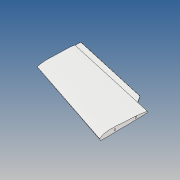
# Autodesk Inventor part: wing_r
Saved by Autodesk Inventor 2019.4 (Build 234330000, 330)
## iProperties
Part Number: wing_r
Material: GEDA Polyamid
Document SubType Name: Modeling
Designer: Admin
Density: 1.14 g/cm^3
Appearance: GEDA Polyamid A
Mass: 6967.25 g
Surface Area: 6132.4 cm^2
Volume: 6111.62 cm^3
Gewicht: 6,967 kg
G_L: 0
G_H: 0
G_B: 0
InventorVersion: 2019.4
VAULT_Status: in Bearbeitung
Revision: -
Max. Breite: 0
Max. Höhe: 0
Max. Länge: 0
Max. Abmessungen: 0 x 0 x 0
Author: Admin
Autodesk Inventor part; units mm, degrees
note: some values were not read from the file. Left out: dimensions or parameters whose unit could not be read.
ref_plane "XZ Plane" through (0, 0, 0) normal (0, 1, 0) x (-1, 0, 0)
ref_plane "XY Plane" through (0, 0, 0) normal (0, 0, 1) x (1, 0, 0)
sketch "Skizze1" plane through (0, 0, 0) normal (1, 0, 0) x (0, 1, 0)
  line L0 (190, 0) -> (-190, 0) construction
  line L1 (190, 4) -> (190, -4)
  arc A0 (-187.5, 0) -> (-191.5, -2) centre (-190, 0) ccw
  line L2 (175, 4) -> (175, -4) construction
  line L3 (160, 4) -> (160, -4) construction
  line L4 (145, 4) -> (145, -4) construction
  line L5 (130, 4) -> (130, -4) construction
  line L6 (115, 4) -> (115, -4) construction
  line L7 (100, 4) -> (100, -4) construction
  line L8 (85, 4) -> (85, -4) construction
  line L9 (70, 4) -> (70, -4) construction
  line L10 (55, 4) -> (55, -4) construction
  line L11 (40, 4) -> (40, -4) construction
  line L12 (25, 4) -> (25, -4) construction
  line L13 (10, 4) -> (10, -4) construction
  line L14 (-5, 4) -> (-5, -4) construction
  line L15 (-20, 4) -> (-20, -4) construction
  line L16 (-35, 4) -> (-35, -4) construction
  line L17 (-50, 4) -> (-50, -4) construction
  line L18 (-65, 4) -> (-65, -4) construction
  line L19 (-80, 4) -> (-80, -4) construction
  line L20 (-95, 4) -> (-95, -4) construction
  line L21 (-110, 4) -> (-110, -4) construction
  line L22 (-125, 4) -> (-125, -4) construction
  line L23 (-140, 4) -> (-140, -4) construction
  line L24 (-155, 4) -> (-155, -4) construction
  line L25 (-170, 4) -> (-170, -4) construction
  line L26 (-185, 4) -> (-185, -4) construction
  spline S0 degree 4 poles (190, 4) (180.693439, 6.175746) (167.34996, 4.728291) (150.73157, 10.619858) (130.00496, 11.534843) (114.926902, 11.944736) (100.09619, 16.366817) (84.995798, 15.753856) (70.031226, 18.172852) (54.977291, 16.655954) (40.010267, 18.831213) (25.003216, 19.470312) (9.999425, 20.120884) (-5.040619, 20.086873) (-19.992496, 22.481196) (-35.017169, 23.283401) (-49.952902, 25.816018) (-64.98949, 26.287803) (-79.991443, 26.127368) (-95.012267, 26.106112) (-109.998953, 26.333155) (-125.124156, 25.693834) (-140.013163, 23.593011) (-155.512337, 21.607881) (-170.0048, 17.338261) (-185.503829, 8.402663) (-188.41231, 4.315767) (-191.5, 2) knots 0 0 0 0 0 0.09690064 0.13564282 0.17442327 0.21313723 0.25184679 0.29053946 0.32917292 0.36780551 0.40642935 0.44505686 0.48369769 0.5223518 0.5610367 0.59972399 0.63838411 0.67702152 0.71562525 0.75422897 0.79286639 0.8315655 0.87050916 0.91018421 0.94746519 1 1 1 1 1
  spline S1 degree 4 poles (190, -4) (180.868607, -8.834605) (167.577093, -7.226631) (150.689794, -8.852336) (129.995932, -9.178584) (115.001025, -9.754105) (100.002885, -10.945984) (84.995429, -9.903483) (69.98651, -10.740277) (55.016309, -12.364457) (40.002357, -12.276351) (24.998782, -13.199765) (10.004392, -11.905004) (-5.001206, -12.101759) (-19.99952, -11.682496) (-35.010481, -11.676294) (-49.996154, -12.753996) (-64.995176, -13.619785) (-79.998423, -13.218732) (-95.007384, -14.395601) (-109.969814, -13.845247) (-125.092444, -13.647586) (-139.768513, -15.101878) (-155.531963, -14.748192) (-169.353489, -12.273677) (-188.456026, -16.245187) (-187.710507, -4.84212) (-191.5, -2) knots 0 0 0 0 0 0.09710576 0.13572651 0.17434907 0.21296785 0.25158844 0.29021826 0.32884607 0.36747425 0.40610163 0.44471606 0.48332881 0.52194087 0.56055673 0.59917667 0.63779642 0.67641887 0.71503441 0.75364539 0.79226218 0.83087751 0.86949779 0.90817124 0.94562322 1 1 1 1 1
  point P0 (0, 0)
  point P1 (0, 0)
  point P2 (175, 5.762055)
  point P3 (160, 7.568582)
  point P4 (145, 10.260397)
  point P5 (130, 11.485616)
  point P6 (115, 12.742364)
  point P7 (100, 15.367746)
  point P8 (85, 16.347768)
  point P9 (70, 17.391401)
  point P10 (55, 17.391401)
  point P11 (40, 18.529054)
  point P12 (25, 19.467026)
  point P13 (10, 19.988015)
  point P14 (-5, 20.572417)
  point P15 (-20, 22.167853)
  point P16 (-35, 23.6255)
  point P17 (-50, 25.402848)
  point P18 (-65, 26.154606)
  point P19 (-80, 26.154606)
  point P20 (-95, 26.154606)
  point P21 (-110, 26.154606)
  point P22 (-125, 25.402848)
  point P23 (-140, 23.6255)
  point P24 (-155, 21.215098)
  point P25 (-170, 16.347768)
  point P26 (-185, 7.568582)
  point P27 (175, -7.682008)
  point P28 (160, -8.150675)
  point P29 (145, -8.783576)
  point P30 (130, -9.246912)
  point P31 (115, -9.874385)
  point P32 (100, -10.498641)
  point P33 (85, -10.281472)
  point P34 (70, -10.900212)
  point P35 (55, -12.02171)
  point P36 (40, -12.471703)
  point P37 (25, -12.755718)
  point P38 (10, -12.200497)
  point P39 (-5, -11.98159)
  point P40 (-20, -11.767642)
  point P41 (-35, -11.8968)
  point P42 (-50, -12.710546)
  point P43 (-65, -13.366077)
  point P44 (-80, -13.53146)
  point P45 (-95, -14.049831)
  point P46 (-110, -13.916712)
  point P47 (-125, -13.979079)
  point P48 (-140, -14.733207)
  point P49 (-155, -14.367191)
  point P50 (-170, -13.675353)
  point P51 (-185, -11.438548)
  dimension "d0" = 380
  dimension "d1" = 8
  dimension "d2" = 5
  dimension "d3" = 15
  dimension "d6" = 15
  dimension "d11" = 1.5
  constraints: 54 end point, 51 vertical alignment, 3 point on circle, 2 coincident, 2 horizontal, 2 midpoint, 2 vertical, 1 centre point, 1 point on line, 129 other
  measures "d0" distance of L0.start L0.end
  measures "d1" distance of L1.start L1.end
  measures "d2" diameter of A0
  measures "d3" distance between parallel lines of L1 L2
  measures "d6" distance of L2.start L3.start
  measures "d11" horizontal distance of L0.end point (-191.5, 2)
ref_plane "Arbeitsebene1" through (-750, 0, 0) normal (1, 0, 0) x (0, 1, 0)
sketch "Skizze2" plane through (-750, 0, 0) normal (1, 0, 0) x (0, 1, 0)
  line L0 (190, 0) -> (-190, 0) construction
  line L1 (60, 0) -> (360, 0) construction
  arc A0 (62.5, 0) -> (58.8, -2.193171) centre (60, 0) ccw
  line L2 (360, 2.5) -> (360, -2.5)
  line L3 (345, 4.297808) -> (345, -3.702192) construction
  line L4 (330, 4.297808) -> (330, -3.702192) construction
  line L5 (315, 4.297808) -> (315, -3.702192) construction
  line L6 (300, 4.297808) -> (300, -3.702192) construction
  line L7 (285, 4.297808) -> (285, -3.702192) construction
  line L8 (270, 4.297808) -> (270, -3.702192) construction
  line L9 (255, 4.297808) -> (255, -3.702192) construction
  line L10 (240, 4.297808) -> (240, -3.702192) construction
  line L11 (225, 4.297808) -> (225, -3.702192) construction
  line L12 (210, 4.297808) -> (210, -3.702192) construction
  line L13 (195, 4.297808) -> (195, -3.702192) construction
  line L14 (180, 4.297808) -> (180, -3.702192) construction
  line L15 (165, 4.297808) -> (165, -3.702192) construction
  line L16 (150, 4.297808) -> (150, -3.702192) construction
  line L17 (135, 4.297808) -> (135, -3.702192) construction
  line L18 (120, 4.297808) -> (120, -3.702192) construction
  line L19 (105, 4.297808) -> (105, -3.702192) construction
  line L20 (90, 4.297808) -> (90, -3.702192) construction
  line L21 (75, 4.297808) -> (75, -3.702192) construction
  spline S0 degree 4 poles (360, 2.5) (350.67805, 4.323905) (337.609234, 7.235216) (320.680845, 8.204256) (300.010588, 9.258039) (284.996502, 9.310774) (270.000986, 10.143319) (255.003303, 10.806812) (240.001346, 11.085943) (225.002545, 11.730684) (209.99756, 11.397248) (194.994678, 11.673037) (179.988937, 12.100357) (165.010405, 13.575452) (150.002171, 13.825659) (134.988959, 14.618808) (119.963668, 13.141728) (104.915431, 12.836982) (87.67454, 9.184692) (74.914131, 7.802516) (64.293652, 5.199039) (58.8, 2.193171) knots 0 0 0 0 0 0.12504391 0.17487719 0.22465944 0.27443145 0.32420033 0.37396949 0.42373293 0.47349157 0.5232527 0.57302623 0.62280466 0.67258337 0.72236578 0.77215061 0.82200605 0.87194651 0.92268931 1 1 1 1 1
  spline S1 degree 4 poles (360, -2.5) (350.77534, -6.061526) (337.56093, -5.704954) (320.649502, -5.267038) (300.00373, -6.649289) (285.004518, -7.411394) (270.001441, -6.855703) (254.999663, -6.992883) (240.000724, -7.339574) (224.999903, -7.300669) (209.999178, -7.096315) (195.000347, -7.143197) (179.99421, -6.487466) (165.006798, -7.778904) (149.996262, -7.502328) (135.008842, -7.180225) (119.973817, -7.827335) (105.010088, -6.49204) (87.665847, -7.546544) (75.027951, -6.323751) (64.237622, -5.168382) (58.8, -2.193171) knots 0 0 0 0 0 0.12506293 0.1749096 0.22475593 0.2746018 0.32444027 0.37427463 0.42410887 0.47394336 0.52377738 0.57361618 0.62345479 0.67329333 0.72313169 0.77296861 0.82280561 0.8726516 0.92318104 1 1 1 1 1
  point P0 (0, 0)
  point P1 (345, 5.381586)
  point P2 (330, 7.414984)
  point P3 (315, 8.476148)
  point P4 (300, 9.115486)
  point P5 (285, 9.466863)
  point P6 (270, 10.110039)
  point P7 (255, 10.729328)
  point P8 (240, 11.156718)
  point P9 (225, 11.534555)
  point P10 (210, 11.518841)
  point P11 (195, 11.707994)
  point P12 (180, 12.310051)
  point P13 (165, 13.33104)
  point P14 (150, 13.926865)
  point P15 (135, 14.162575)
  point P16 (120, 13.368433)
  point P17 (105, 12.264687)
  point P18 (90, 9.916387)
  point P19 (75, 7.41217)
  point P20 (345, -5.429767)
  point P21 (330, -5.647567)
  point P22 (315, -5.834087)
  point P23 (300, -6.599319)
  point P24 (285, -7.144916)
  point P25 (270, -6.993534)
  point P26 (255, -7.036243)
  point P27 (240, -7.261369)
  point P28 (225, -7.266713)
  point P29 (210, -7.145089)
  point P30 (195, -7.006223)
  point P31 (180, -6.877035)
  point P32 (165, -7.465421)
  point P33 (150, -7.491508)
  point P34 (135, -7.371819)
  point P35 (120, -7.434014)
  point P36 (105, -6.942805)
  point P37 (90, -7.027191)
  point P38 (75, -6.212014)
  point P39 (210, 0.297808)
  dimension "d13" = 250
  dimension "d14" = 300
  dimension "d15" = 5
  dimension "d16" = 5
  dimension "d17" = 8
  dimension "d18" = 15
  dimension "d21" = 15
  dimension "d26" = 1.2
  constraints: 42 end point, 39 vertical alignment, 3 point on circle, 2 horizontal, 2 midpoint, 2 point on line, 2 vertical, 1 centre point, 1 coincident, 99 other
  measures "d13" distance of L0.end L1.start
  measures "d14" distance of L1.end L1.start
  measures "d15" diameter of A0
  measures "d16" distance of L2.start L2.end
  measures "d17" distance of L3.start L3.end
  measures "d18" distance between parallel lines of L2 L3
  measures "d21" distance of L3.start L4.start
  measures "d26" horizontal distance of L1.start point (58.8, 2.193)
loft "Erhebung1" add profiles "Skizze1", "Skizze2"
sketch "Skizze4" plane through (0, 190, 4) normal (1, 0, 0) x (0, 0, -1)
  circle A0 centre (-1, -260) radius 7
  circle A1 centre (-1, -90) radius 7
  line L0 (-1, -260) -> (-1, -90) construction
  arc A2 (2, -381.5) -> (6, -381.5) centre (4, -380) ccw projected
  point P0 (-1, -190)
  dimension "d36" = 14
  dimension "d40" = 170
  dimension "d59" = 5
  dimension "d60" = 120
  constraints: 2 centre point, 2 end point, 1 equal radius, 1 point on line, 1 vertical
  measures "d36" diameter of A0
  measures "d40" distance of L0.start L0.end
  measures "d59" distance from line of A2.centre L0
  measures "d60" vertical distance of A2.centre L0.start
extrude "Extrusion1" cut sketch "Skizze4" against normal blind 120
sketch "Skizze5" plane through (-750, 209.456692, 6.94731) normal (-1, 0, 0) x (0, 0.1920162, 0.9813918)
  line L0 (24.542202, 148.595917) -> (19.635243, 149.555998)
  line L1 (24.542202, 148.595917) -> (33.182931, 192.758546)
  line L2 (33.182931, 192.758546) -> (32.201539, 192.950562)
  line L3 (32.201539, 192.950562) -> (20.72552, 153.320997)
  line L4 (20.72552, 153.320997) -> (24.542202, 148.595917)
  point P0 (-47.037112, -204.225074)
  dimension "d41" = 1
  dimension "d42" = 45
  dimension "d43" = 50
  dimension "d44" = 90
  constraints: 8 end point, 1 parallel, 1 point on line
  measures "d41" distance of L1.end L2.end
  measures "d42" distance between parallel lines of L0 L2
  measures "d43" angle of L1 L4
  measures "d44" angle of L0 L1
sketch3d "3D-Skizze1"
  line L0 (-750, 360, 2.5) -> (0, 190, 4)
sweep "Sweeping1" add profiles "Skizze5" path "3D-Skizze1"
sketch "Skizze6" plane through (-750, 360, 2.5) normal (-0.002, 0, 0.999998) x (0.999998, 0, 0.002)
  line L0 (0, 0) -> (0, 45)
  line L1 (750.0015, -170) -> (0, 0) construction
  line L2 (750.0015, -125) -> (750.0015, -170)
  line L3 (0, 45) -> (750.0015, -125) construction
  line L4 (750.0015, -125) -> (750.0015, -170)
  line L5 (615.393645, -92.438213) -> (752.0015, -123.402598)
  line L6 (752.0015, -123.402598) -> (752.0015, -170.453332)
  line L7 (615.393645, -92.438213) -> (650.0015, -147.333379)
  line L8 (750.0015, -170) -> (0, 0)
  line L9 (752.0015, -170.453332) -> (650.0015, -147.333379)
  line L10 (0, 0) -> (3, -0.679999)
  line L11 (3, -0.679999) -> (3, 50.453332)
  line L12 (3, 50.453332) -> (-2, 50.453332)
  line L13 (-2, 50.453332) -> (-2, 0.453332)
  line L14 (-2, 0.453332) -> (0, 0)
  line L15 (-0.002, 45) -> (749.9995, -125)
  point P0 (749.9935, -360)
  point P1 (749.9855, -170)
  dimension "d47" = 100
  dimension "d53" = 2
  dimension "d54" = 45
  dimension "d55" = 2
  dimension "d56" = 3
  dimension "d57" = 5
  dimension "d58" = 50
  constraints: 18 end point, 3 point on line, 2 perpendicular, 2 vertical, 1 collinear, 1 parallel
  measures "d47" horizontal distance of L1.start L7.end
  measures "d53" distance between parallel lines of L3 L5
  measures "d54" angle of L1 L7
  measures "d55" distance between parallel lines of L2 L6
  measures "d56" distance between parallel lines of L0 L11
  measures "d57" distance of L11.end L12.end
  measures "d58" distance of L12.end L13.end
extrude "Extrusion2" cut sketch "Skizze6" against normal through all contours L14 L13 L12 L11 L15 L0 | L0 L15 L11 L8 | L7 L15 L2 L8 | L7 L5 L6 L9 L2 L15
equation "\"G_L\" = 0"
equation "\"G_H\" = 0"
equation "\"G_B\" = 0"
